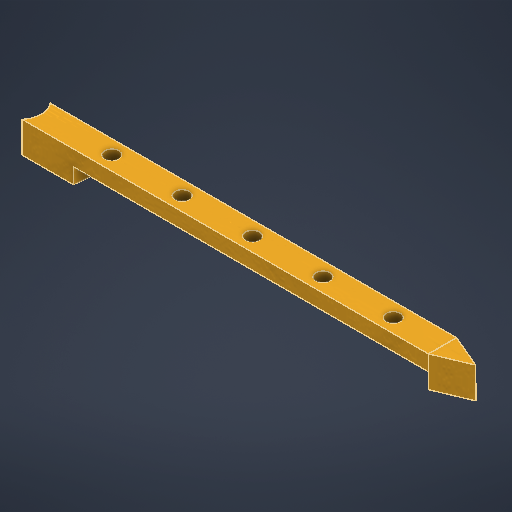
# Autodesk Inventor part: measuring_triangle
Saved by Autodesk Inventor 2026.1 (Build 301233000, 233)
## iProperties
Created: 2025-12-25
Part Number: measuring_triangle
Material: Generic
Document SubType Name: Modeling
Designer: emanuel
Density: 1 g/cm^3
Appearance: Weld - Brass
Author: emanuel
Autodesk Inventor part; units mm, degrees
ref_plane "YZ Plane" through (0, 0, 0) normal (1, 0, 0) x (0, 1, 0)
ref_plane "XZ Plane" through (0, 0, 0) normal (0, 1, 0) x (-1, 0, 0)
ref_plane "XY Plane" through (0, 0, 0) normal (0, 0, 1) x (1, 0, 0)
sketch "Sketch1" plane through (0, 0, 0) normal (0, 1, 0) x (-1, 0, 0)
  circle A0 centre (0, 0) radius 3.1
  circle A1 centre (0, 0) radius 9.85
  circle A2 centre (0, 0) radius 60.1
  circle A3 centre (0, 0) radius 64.85
  line L0 (0, 0) -> (-64.85, 0)
  line L1 (-36.1453, 0) -> (-36.1453, -2)
  line L2 (-36.1453, -2) -> (-36.1453, 2)
  line L3 (-36.1453, -2) -> (-64.8192, -2)
  line L4 (-64.8192, -2) -> (-64.8192, 2)
  line L5 (-64.8192, 2) -> (-36.1453, 2)
  line L6 (-36.1453, 2) -> (-36.1453, -2)
  line L7 (-36.1453, -2) -> (0, -2)
  line L8 (0, -2) -> (0, 2)
  line L9 (0, 2) -> (-36.1453, 2)
  line L10 (-36.1453, 2) -> (-36.1453, -2)
  line L11 (-60.0667, -2) -> (-64.85, 0)
  line L12 (-60.0667, 2) -> (-64.85, 0)
  point P0 (-64.8192, -0.0129)
  point P1 (-64.8192, 0.0129)
  point P2 (-9.6448, -2)
  point P3 (-2.3685, -2)
  point P4 (-2.3685, 2)
  point P5 (-9.6448, 2)
  dimension "d15" = 6.2
  dimension "d16" = 19.7
  dimension "d17" = 120.2
  dimension "d18" = 129.7
  dimension "d19" = 2
  dimension "d20" = 4
  constraints: 26 end point, 5 point on line, 4 centre point, 4 parallel, 4 point on circle, 3 coincident, 3 horizontal, 3 perpendicular
  measures "d15" diameter of A0
  measures "d16" diameter of A1
  measures "d17" diameter of A2
  measures "d18" diameter of A3
  measures "d19" distance of L1.start L1.end
  measures "d20" distance of L1.end L2.end
extrude "Extrusion1" add sketch "Sketch1" along normal blind 2.2 contours A0 L0 A1 L9 | L7 A1 L0 A0 | A2 L0 L4 L12 | L11 L4 L0 A2
sketch "Sketch3" plane through (0, 2.2, 0) normal (0, 1, 0) x (1, 0, 0)
  circle A0 centre (0, 0) radius 3.1
  circle A1 centre (0, 0) radius 9.85
  circle A2 centre (0, 0) radius 60.1
  line L0 (9.6448, 2) -> (2.3685, 2) projected
  line L1 (2.3685, 2) -> (60.0667, 2)
  line L2 (60.0667, 2) -> (60.0667, -2)
  line L3 (60.0667, -2) -> (2.3685, -2)
  line L4 (2.3685, -2) -> (2.3685, 2)
  line L5 (60.0667, -2) -> (64.8192, -0.0129) projected
  line L6 (60.0667, 2) -> (64.8192, -0.0129)
  line L7 (64.8192, -0.0129) -> (60.0667, -2)
  point P0 (2.3685, -2)
  constraints: 12 end point, 3 coincident, 3 equal length, 1 horizontal, 1 perpendicular, 7 other
extrude "Extrusion3" add sketch "Sketch3" along normal blind 2.2 contours A0 L0 A1 L3 | L1 L2 L3 A1 | L6 L5 A2 picked at (5.2914, -0.6855)
sketch "Sketch4" plane through (0, 4.4, 0) normal (0, 1, 0) x (1, 0, 0)
  arc A0 (2.3685, -2) -> (2.3685, 2) centre (0, 0) ccw projected
  line L0 (3.1, 0) -> (13.1, 0)
  line L1 (13.1, 0) -> (23.1, 0)
  line L2 (23.1, 0) -> (33.1, 0)
  line L3 (33.1, 0) -> (43.1, 0)
  line L4 (43.1, 0) -> (53.1, 0)
  circle A1 centre (13.1, 0) radius 1
  circle A2 centre (23.1, 0) radius 1
  circle A3 centre (33.1, 0) radius 1
  circle A4 centre (43.1, 0) radius 1
  circle A5 centre (53.1, 0) radius 1
  dimension "d23" = 10
  dimension "d24" = 10
  dimension "d25" = 10
  dimension "d26" = 10
  dimension "d27" = 10
  dimension "d28" = 2
  dimension "d29" = 2
  dimension "d30" = 2
  dimension "d31" = 2
  dimension "d32" = 2
  constraints: 10 end point, 5 centre point, 5 coincident, 4 point on line, 1 horizontal, 1 point on circle
  measures "d23" distance of L0.start L0.end
  measures "d24" distance of L0.end L1.end
  measures "d25" distance of L1.end L2.end
  measures "d26" distance of L2.end L3.end
  measures "d27" distance of L3.end L4.end
  measures "d28" diameter of A1
  measures "d29" diameter of A2
  measures "d30" diameter of A3
  measures "d31" diameter of A4
  measures "d32" diameter of A5
extrude "Extrusion4" cut sketch "Sketch4" against normal blind 2.2
body "Solid1"
